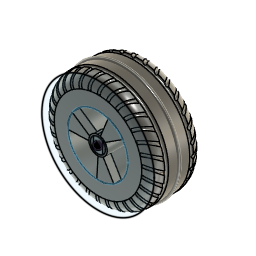
final__tyre_ (Autodesk Fusion 360 design; units mm, degrees)
Autodesk Fusion 360 part; units mm, degrees
note: some values were not read from the file. Chosen so that the rebuilt part matches the saved one: which face or edge a step refers to.
sketch "Sketch1" plane through (0, 0, 0) normal (0, 1, 0) x (1, 0, 0)
  circle A0 centre (0, 0) radius 22.5
  circle A1 centre (0, 0) radius 12
  dimension "d1" = 45
  constraint coincident A0.centre A1.centre
  measures "d1" diameter of A0
extrude "Extrude1" add sketch "Sketch1" along normal blind 10 makes body 1
sketch "Sketch2" plane through (0, 0, 0) normal (0, 1, 0) x (1, 0, 0)
  circle A0 centre (0, 0) radius 17.5
  circle A1 centre (0, 0) radius 22.5
  dimension "d4" = 35
  dimension "d5" = 45
  constraint coincident A0.centre A1.centre
  constraint concentric A0 A1
  measures "d4" diameter of A0
  measures "d5" diameter of A1
fillet "Fillet1" radius 5 1 edges at (-20.9774, 0, 8.1363) on bodies 1
sketch "Sketch3" plane through (0, 0, 0) normal (1, 0, 0) x (0, 1, 0)
  line L0 (5, 22.5) -> (5, -22.5)
  line L1 (0, -17.5) -> (0, 17.5)
  arc A0 (5, 22.5) -> (0, 17.5) centre (5, 17.5) ccw
  constraint tangent L1 A0
  constraint coincident L0.start A0.start
  constraint coincident L1.end A0.end
pipe "Pipe1" add diameter 1.5 path "Sketch3" along A0 separate body makes body 2
move_body "Move1" bodies 2 to x (0.866025, -0.5, 0) y (0.5, 0.866025, 0) z (0, 0, 1) at (0.2745, -0.4755, 0)
move_face "OffsetFaces1" offset 1.2 1 faces at (2.5043, 4.0106, 22.2441) on bodies 2
pipe "Pipe2" cut diameter 1.5 along 1 edges at (-22.5, 5, 0) on bodies 1 bodies 1 2
pattern_circular "C-Pattern1" count 30 over 360 about axis through (0, 0, 0) along (0, 1, 0) of bodies 2 makes body 3 at (6.7501, 4.0959, 21.1183) makes body 4 at (11.017, 4.0862, 19.173) makes body 5 at (14.7625, 4.0862, 16.4632) makes body 6 at (17.8627, 4.0859, 13.0327) makes body 7 at (20.2093, 4.0955, 9.1116) makes body 8 at (21.6607, 4.0952, 4.7087) makes body 9 at (22.1648, 4.0949, 0.1008) makes body 10 at (21.7059, 4.0956, -4.507) makes body 11 at (20.2182, 4.086, -8.9531) makes body 12 at (17.9168, 4.0863, -12.9607) makes body 13 at (14.8291, 4.0861, -16.4025) makes body 14 at (11.1769, 4.0959, -19.147) makes body 15 at (6.9486, 4.0954, -21.0507) makes body 16 at (2.416, 4.0947, -22.0319) makes body 17 at (-2.2157, 4.0951, -22.055) makes body 18 at (-6.7501, 4.0959, -21.1183) makes body 19 at (-11.017, 4.0862, -19.173) makes body 20 at (-14.7625, 4.0862, -16.4632) makes body 21 at (-17.8627, 4.0859, -13.0327) makes body 22 at (-20.2093, 4.0955, -9.1116) makes body 23 at (-21.6607, 4.0952, -4.7087) makes body 24 at (-22.1648, 4.0949, -0.1008) makes body 25 at (-21.7059, 4.0956, 4.507) makes body 26 at (-20.2182, 4.086, 8.9531) makes body 27 at (-17.9168, 4.0863, 12.9607) makes body 28 at (-14.8291, 4.0861, 16.4025) makes body 29 at (-11.1769, 4.0959, 19.147) makes body 30 at (-6.9486, 4.0954, 21.0507) makes body 31 at (-2.416, 4.0947, 22.0319)
combine "Combine1" operation cut target body 1 tool bodies 2 3 4 8 5 6 7 9 11 10 12 13 15 14 16 17 18 19 20 21 23 22 24 25 26 27 28 29 31 30
mirror "Mirror1" about plane through (0, 10, 0) normal (0, 1, 0) of bodies 1 merged
sketch "Sketch4" plane through (0, 0, 0) normal (1, 0, 0) x (0, 1, 0)
pipe "Pipe3" add diameter 1.5 path "Sketch2" along A1 separate body makes body 32
move_body "Move2" bodies 32 to x (1, 0, 0) y (0, 1, 0) z (0, 0, 1) at (0, 10, 0)
sketch "Sketch5" plane through (0, 0, 0) normal (0, 1, 0) x (1, 0, 0)
  circle A0 centre (0, 0) radius 3
  circle A1 centre (0, 0) radius 3.7013
  dimension "d26" = 6
  constraint coincident A0.centre A1.centre
  constraint concentric A0 A1
  measures "d26" diameter of A0
extrude "Extrude2" add sketch "Sketch5" along normal blind 20 separate body makes body 33
sketch "Sketch6" plane through (0, 0, 0) normal (0, 1, 0) x (1, 0, 0)
  line L0 (0.9048, -3.4992) -> (4.1427, -11.4741)
  line L1 (4.1427, -11.4741) -> (7, -10)
  line L2 (7, -10) -> (8.5799, -8.6259)
  line L3 (8.5799, -8.6259) -> (10, -7)
  line L4 (10, -7) -> (2.7036, -2.3299)
  line L5 (2, 3) -> (6.3318, 10.3028)
  line L6 (6.3318, 10.3028) -> (4.1659, 11.2628)
  line L7 (4.1659, 11.2628) -> (2, 12)
  line L8 (2, 12) -> (-0.5032, 12)
  line L9 (-0.5032, 12) -> (-0.0041, 3.5446)
  line L10 (-3.6412, 0.275) -> (-12, 0.5)
  line L11 (-12, 0.5) -> (-12.0603, -1.7397)
  line L12 (-12.0603, -1.7397) -> (-11.5, -4)
  line L13 (-11.5, -4) -> (-10.3428, -6.3005)
  line L14 (-10.3428, -6.3005) -> (-3.2381, -1.4381)
  spline S0 degree 5 poles (-3.2381, -1.4381) (-3.2329, -1.4747) (-3.2184, -1.5494) (-3.1848, -1.6663) (-3.116, -1.8318) (-2.9892, -2.0544) (-2.821, -2.2911) (-2.612, -2.5376) (-2.3644, -2.786) (-2.0824, -3.0257) (-1.7708, -3.2444) (-1.4346, -3.4303) (-1.0785, -3.5732) (-0.7062, -3.6663) (-0.3205, -3.7067) (0.0768, -3.694) (0.403, -3.6417) (0.6522, -3.5794) (0.8202, -3.5276) (0.9048, -3.4992) knots 0 0 0 0 0 0 0.066667 0.133333 0.2 0.266667 0.333333 0.4 0.466667 0.533333 0.6 0.666667 0.733333 0.8 0.866667 0.933333 1 1 1 1 1 1
  spline S1 degree 5 poles (2.7036, -2.3299) (2.7122, -2.3218) (2.7303, -2.3048) (2.7602, -2.2775) (2.8058, -2.2374) (2.872, -2.18) (2.947, -2.1131) (3.0295, -2.0318) (3.1176, -1.9292) (3.209, -1.7987) (3.3007, -1.6358) (3.3898, -1.4401) (3.4731, -1.2163) (3.5473, -0.972) (3.6094, -0.7161) (3.6563, -0.4573) (3.6856, -0.2027) (3.6949, 0.0447) (3.6826, 0.285) (3.6475, 0.5205) (3.5895, 0.7543) (3.509, 0.9894) (3.4078, 1.2271) (3.2887, 1.4662) (3.1553, 1.7033) (3.0118, 1.9337) (2.8623, 2.1524) (2.7107, 2.3541) (2.5601, 2.5347) (2.4127, 2.6913) (2.2697, 2.8225) (2.1593, 2.9066) (2.0787, 2.9579) (2.0261, 2.9868) (2, 3) knots 0 0 0 0 0 0 0.033333 0.066667 0.1 0.133333 0.166667 0.2 0.233333 0.266667 0.3 0.333333 0.366667 0.4 0.433333 0.466667 0.5 0.533333 0.566667 0.6 0.633333 0.666667 0.7 0.733333 0.766667 0.8 0.833333 0.866667 0.9 0.933333 0.966667 1 1 1 1 1 1
  spline S2 degree 5 poles (-3.6412, 0.275) (-3.6402, 0.298) (-3.6372, 0.3452) (-3.6296, 0.42) (-3.6134, 0.5274) (-3.5829, 0.6747) (-3.5423, 0.8343) (-3.4918, 1.0049) (-3.4321, 1.1842) (-3.3636, 1.3691) (-3.2866, 1.5565) (-3.2001, 1.7434) (-3.1019, 1.9282) (-2.9884, 2.1101) (-2.8548, 2.2895) (-2.697, 2.4667) (-2.5123, 2.6416) (-2.3003, 2.8133) (-2.0644, 2.9792) (-1.8106, 3.1352) (-1.5468, 3.2768) (-1.2816, 3.3992) (-1.0231, 3.498) (-0.7782, 3.5694) (-0.5515, 3.6114) (-0.3453, 3.6226) (-0.1978, 3.6069) (-0.0971, 3.5811) (-0.0343, 3.5578) (-0.0041, 3.5446) knots 0 0 0 0 0 0 0.04 0.08 0.12 0.16 0.2 0.24 0.28 0.32 0.36 0.4 0.44 0.48 0.52 0.56 0.6 0.64 0.68 0.72 0.76 0.8 0.84 0.88 0.92 0.96 1 1 1 1 1 1
  point P0 (-2.7512, -2.3677)
  point P1 (-1.2463, -3.4992)
  point P2 (2.9064, -2.1488)
  point P3 (3.2687, -1.6877)
  point P4 (3.6639, -0.3704)
  point P5 (3.5, 1)
  point P6 (2.7036, 2.3581)
  point P7 (-3.5324, 0.8637)
  point P8 (-3.203, 1.731)
  point P9 (-2.4785, 2.6642)
  point P10 (-1, 3.5)
  constraint horizontal L8
  constraint perpendicular L10 L11
extrude "Extrude3" add sketch "Sketch6" along normal blind 3 separate body makes body 34
sketch "Sketch7" plane through (0, 0, 0) normal (0, 1, 0) x (1, 0, 0)
  circle A0 centre (0, 0) radius 3
  line L0 (1.8114, -2.3914) -> (1.8114, 2.3914)
  line L1 (-1.8114, -2.3914) -> (-1.8114, 2.3914)
  constraint coincident A0.centre origin
  constraint coincident A0 L0.start
  constraint coincident A0 L0.end
  constraint vertical L0
  constraint coincident A0 L1.start
  constraint coincident A0 L1.end
  constraint parallel L0 L1
extrude "Extrude4" cut sketch "Sketch7" along normal blind 20 contours A0 L0 | A0 L1 bodies 34
sketch "Sketch8" plane through (0, 0, 0) normal (0, 1, 0) x (1, 0, 0)
  circle A0 centre (0, 0) radius 3
  line L0 (-1.8728, -2.3437) -> (-1.8728, 2.3437)
  line L1 (1.8728, -2.3437) -> (1.8728, 2.3437)
  dimension "d33" = 6
  constraint coincident A0.centre origin
  constraint coincident A0 L0.start
  constraint coincident A0 L0.end
  constraint vertical L0
  constraint coincident A0 L1.start
  constraint coincident A0 L1.end
  constraint parallel L0 L1
  measures "d33" diameter of A0
extrude "Extrude5" add sketch "Sketch8" along normal blind 20 contours A0 L1 | A0 L0 bodies 33 34
sketch "Sketch9" plane through (0, 0, 0) normal (0, 1, 0) x (1, 0, 0)
  circle A0 centre (0, 0) radius 3.7
  circle A1 centre (0, 0) radius 3
  dimension "d36" = 6
  constraint coincident A0.centre A1.centre
  constraint concentric A0 A1
  measures "d36" diameter of A1
extrude "Extrude6" add sketch "Sketch9" along normal blind 24 separate body makes body 35
move_face "MoveFace1" to x (1, 0, 0) y (0, 1, 0) z (0, 0, 1) at (0, -4, 0) 1 faces at (3.6816, 8, 0.3684) on bodies 35
sketch "Sketch10" plane through (0, 0, 0) normal (0, 1, 0) x (1, 0, 0)
  circle A0 centre (0, 0) radius 3
  dimension "d39" = 6
  constraint coincident A0.centre origin
  measures "d39" diameter of A0
sketch "Sketch11" plane through (0, 0, 0) normal (0, 1, 0) x (1, 0, 0)
